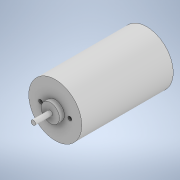
# Autodesk Inventor part: RD008_モータ(DMN29)
Saved by Autodesk Inventor 2021 (Build 250183000, 183)
## iProperties
Created: 2020-11-01
Part Number: RD008_モータ(DMN29)
Material: 一般
Document SubType Name: Modeling
Designer: ryusei
Density: 1 g/cm^3
Appearance: 既定
Author: ryusei
Autodesk Inventor part; units mm, degrees
ref_plane "YZ Plane" through (0, 0, 0) normal (1, 0, 0) x (0, 1, 0)
ref_plane "XZ Plane" through (0, 0, 0) normal (0, 1, 0) x (-1, 0, 0)
ref_plane "XY Plane" through (0, 0, 0) normal (0, 0, 1) x (1, 0, 0)
sketch "スケッチ1" plane through (0, 0, 0) normal (0, 0, 1) x (1, 0, 0)
  circle A0 centre (0, 0) radius 14.5
  dimension "d0" = 29
  constraints: 1 centre point, 1 coincident
  measures "d0" diameter of A0
extrude "押し出し1" add sketch "スケッチ1" along normal blind 50
sketch "スケッチ2" plane through (0, 0, 50) normal (0, 0, 1) x (1, 0, 0)
  circle A0 centre (0, 0) radius 5
  dimension "d3" = 10
  constraints: 1 centre point, 1 coincident
  measures "d3" diameter of A0
extrude "押し出し2" add sketch "スケッチ2" along normal blind 2.7
sketch "スケッチ3" plane through (0, 0, 52.7) normal (0, 0, 1) x (1, 0, 0)
  circle A0 centre (0, 0) radius 1.25
  dimension "d6" = 2.5
  constraints: 1 centre point, 1 coincident
  measures "d6" diameter of A0
extrude "押し出し3" add sketch "スケッチ3" along normal blind 9.3
sketch "スケッチ4" plane through (0, 0, 50) normal (0, 0, 1) x (1, 0, 0)
  circle A0 centre (0, 0) radius 14.5 projected
  line L0 (0, 14.5) -> (0, -14.5)
  point P0 (-8, 0)
  point P1 (8, 0)
  dimension "d9" = 16
  constraints: 2 end point, 2 point on circle, 1 symmetric about line, 1 vertical
  measures "d9" distance of point (8, 0) point (-8, 0)
hole "穴1" at (-8, 0, 50) at (8, 0, 50) direction (0, 0, -1) diameter 2.1129 depth 3 tip angle 118 thread size "M2.6x0.45" class "6H" standard "ISO Metric profile"
